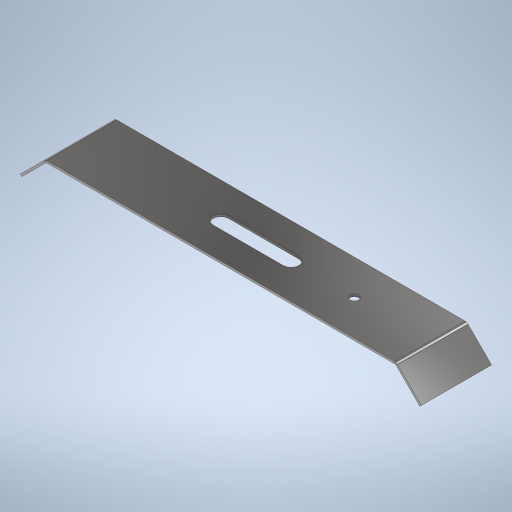
# Autodesk Inventor part: 2309HCMUTE-CDT23_TAY-GAT
Saved by Autodesk Inventor 2023 (Build 270158000, 158)
## iProperties
Created: 2023-10-13
Part Number: 2309HCMUTE-CDT23_TAY-GAT
Material: Stainless Steel
Document SubType Name: Sheet Metal
Designer: havie
Density: 8 g/cm^3
Sheet Metal Rule: Default_mm
Appearance: Steel - Polished
Mass: 345.674 g
Surface Area: 312.291 cm^2
Volume: 43.2092 cm^3
Flat Pattern Width: 5 cm
Flat Pattern Length: 29.8422 cm
Flat Pattern Area: 149.211 cm^2
Sheet Metal Width: 50.000 mm
Sheet Metal Length: 298.422 mm
Sheet Metal Area: 14921.118 mm^2
Author: havie
Autodesk Inventor part; units mm, degrees
ref_plane "YZ Plane" through (0, 0, 0) normal (1, 0, 0) x (0, 1, 0)
ref_plane "XZ Plane" through (0, 0, 0) normal (0, 1, 0) x (-1, 0, 0)
ref_plane "XY Plane" through (0, 0, 0) normal (0, 0, 1) x (1, 0, 0)
sketch "Sketch4" plane through (0, 0, 0) normal (0, 1, 0) x (-1, 0, 0)
  line L0 (125, 25) -> (-125, 25)
  line L1 (-125, 25) -> (-125, -25)
  line L2 (-125, -25) -> (125, -25)
  line L3 (125, -25) -> (125, 25)
  line L4 (125, 25) -> (-125, -25) construction
  line L5 (-125, 25) -> (125, -25) construction
  line L6 (25, 0) -> (-25, 0) construction
  line L7 (25, 5.5) -> (-25, 5.5)
  line L8 (-25, -5.5) -> (25, -5.5)
  arc A0 (25, -5.5) -> (25, 5.5) centre (25, 0) ccw
  arc A1 (-25, 5.5) -> (-25, -5.5) centre (-25, 0) ccw
  point P0 (0, 0)
  point P1 (0, 0)
  dimension "d17" = 250
  dimension "d18" = 50
  dimension "d19" = 50
  dimension "d20" = 11
  measures "d17" distance of L1.end L2.end
  measures "d18" distance of L0.end L1.end
  measures "d19" distance of L8.start L8.end
  measures "d20" distance between parallel lines of L7 L8
extrude "Plate3" add sketch "Sketch4" along normal blind 1.5
sketch "Sketch6" plane through (-123.9393, 0.4393, -25) normal (-0.7071068, 0.7071068, 0) x (-0.7071068, -0.7071068, 0)
  line L0 (0, 50) -> (0, 0)
  line L1 (0, 0) -> (25, 0)
  line L2 (25, 0) -> (25, 50)
  line L3 (25, 50) -> (0, 50)
  constraints: 6 end point, 1 horizontal, 1 perpendicular, 1 vertical
edge flange "Flange3" height 25 angle 45 thickness 1.5 bend radius 1.5 thickness toward (-0.7071068, 0.7071068, 0) relief tear relief width 1.5 relief depth 0.75 corner gap 1.5 corner form 0 edges at (-125, 0, 0) (125, 0, 0) wall of the first edge with corners at (-123.9393, 0.4393, 25) (-123.9393, 0.4393, -25) (-141.617, -17.2383, -25) (-141.617, -17.2383, 25)
bend "Bend3"
corner "Corner3"
sketch "Sketch7" plane through (0, 1.5, 0) normal (0, 1, 0) x (1, 0, 0)
  circle A0 centre (70, 0) radius 3
  point P0 (0, 0)
  dimension "d43" = 70
  dimension "d44" = 6
  constraints: 1 centre point, 1 horizontal alignment
  measures "d43" distance of A0.centre point (0, 0)
  measures "d44" diameter of A0
extrude "Cut2" cut sketch "Sketch7" against normal blind 1.5
equation "\"d41\" = Thickness"
equation "\"d2\" = Thickness"
equation "\"d31\" = BendReliefWidth"
equation "\"d32\" = BendReliefDepth"
equation "\"d33\" = MinimumRemnant"
equation "\"d34\" = TransitionRadius"
equation "\"d37\" = BendRadius"
equation "\"d38\" = CornerReliefSize"
equation "\"d39\" = GapSize"
equation "\"d40\" = JacobiRadiusSize"
equation "\"BendRadius\" = Thickness"
equation "\"BendReliefWidth\" = Thickness"
equation "\"BendReliefDepth\" = 0.5 * Thickness"
equation "\"CornerReliefSize\" = 4 * Thickness"
equation "\"MinimumRemnant\" = 2 * Thickness"
equation "\"TransitionRadius\" = BendRadius"
equation "\"JacobiRadiusSize\" = BendRadius"
equation "\"GapSize\" = Thickness"
equation "\"Thickness\" = 1.5"
body "Solid1"
